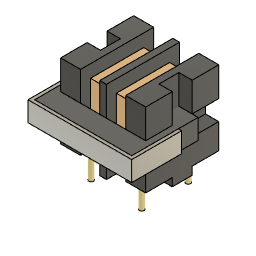
PowerLine_choke v2 (Autodesk Fusion 360 design; units mm, degrees)
Autodesk Fusion 360 part; units mm, degrees
note: some values were not read from the file. Chosen so that the rebuilt part matches the saved one: which bodies a step acts on.
sketch "Sketch1" plane through (0, 0, 0) normal (0, 0, 1) x (1, 0, 0) in component "PowerLine_choke"
  line L0 (10.2, -2) -> (10.2, 9)
  line L1 (-2.6, 9) -> (-2.6, -2)
  line L2 (7.2, 9) -> (7.2, -2)
  line L3 (0.4, 9) -> (0.4, -2)
  circle A0 centre (0, 7) radius 0.35
  circle A1 centre (7.62, 7) radius 0.35
  circle A2 centre (0, 0) radius 0.35
  circle A3 centre (7.62, 0) radius 0.35
  line L4 (3.3, 9) -> (3.3, -2)
  line L5 (4.3, -2) -> (4.3, 9)
  line L6 (0.4, 9) -> (-2.6, 9)
  line L7 (10.2, 9) -> (7.2, 9)
  line L8 (4.3, 9) -> (3.3, 9)
  line L9 (7.2, -2) -> (10.2, -2)
  line L10 (-2.6, -2) -> (0.4, -2)
  line L11 (3.3, -2) -> (4.3, -2)
  line L12 (7.2, -0.5) -> (4.3, -0.5)
  line L13 (3.3, -0.5) -> (0.4, -0.5)
  line L14 (0.4, 7.5) -> (3.3, 7.5)
  line L15 (4.3, 7.5) -> (7.2, 7.5)
  line L16 (10.2, 2) -> (8.2, 2)
  line L17 (-0.6, 2) -> (-2.6, 2)
  line L18 (-2.6, 5) -> (-0.6, 5)
  line L19 (8.2, 5) -> (10.2, 5)
  line L20 (8.2, 5) -> (8.2, 2)
  line L21 (-0.6, 5) -> (-0.6, 2)
  line L22 (-0.6, 5) -> (8.2, 5)
  line L23 (8.2, 2) -> (-0.6, 2)
  line L24 (-0.6, 5) -> (-0.6, 9)
  line L25 (-0.6, 2) -> (-0.6, -2)
  line L26 (8.2, 2) -> (8.2, -2)
  line L27 (8.2, 5) -> (8.2, 9)
  dimension "d1" = 7.62
  dimension "d2" = 7
  dimension "d3" = 12.8
  dimension "d4" = 11
  dimension "d6" = 3
  dimension "d7" = 0.7
  dimension "d8" = 0.7
  dimension "d9" = 0.7
  dimension "d10" = 0.7
  constraint horizontal L10
  constraint vertical L0
  constraint horizontal L7
  constraint vertical L1
  constraint coincident L2.end L10
  constraint perpendicular L2 L10
  constraint perpendicular L3 L10
  constraint coincident L3.start L7
  constraint coincident A2.centre origin
  constraint collinear L6 L7
  constraint collinear L7 L8
  constraint collinear L9 L10
  constraint collinear L10 L11
  constraint horizontal L14
  constraint horizontal L12
  constraint coincident L2 L12.start
  constraint coincident L2 L15.end
  constraint coincident L3 L14.start
  constraint coincident L3 L13.end
  constraint coincident L5 L12.end
  constraint coincident L4 L13.start
  constraint collinear L12 L13
  constraint coincident L4 L14.end
  constraint coincident L5 L15.start
  constraint collinear L14 L15
  constraint horizontal L18
  constraint horizontal L16
  constraint coincident L1 L18.start
  constraint coincident L1 L17.end
  constraint coincident L0 L19.end
  constraint coincident L0 L16.start
  constraint collinear L16 L17
  constraint collinear L18 L19
  constraint perpendicular L16 L20
  constraint perpendicular L17 L21
  constraint perpendicular L20 L22
  constraint perpendicular L21 L23
  constraint coincident L6 L24.end
  constraint perpendicular L6 L24
  constraint perpendicular L23 L25
  constraint coincident L9 L26.end
  constraint perpendicular L9 L26
  constraint coincident L7 L27.end
  constraint perpendicular L7 L27
  measures "d1" distance of A2.centre A3.centre
  measures "d2" distance of A2.centre A0.centre
  measures "d3" distance of L1.end L0.start
  measures "d4" distance of L1.end L1.start
  measures "d6" distance of L1 L3
  measures "d7" diameter of A0
  measures "d8" diameter of A1
  measures "d9" diameter of A2
  measures "d10" diameter of A3
extrude "Extrude1" add sketch "Sketch1" along normal blind 12.4 contours L0 L9 L16 L26 | L2 L9 L23 L26 | L0 L7 L19 L27 | L2 L20 L22 L23 | L2 L7 L22 L27 | L4 L5 L22 L23 | L4 L5 L11 L23 | L4 L5 L8 L22 | L3 L21 L22 L23 | L3 L10 L23 L25 | L3 L6 L22 L24 | L1 L10 L17 L25 | L1 L6 L18 L24 | A0 | A1 | A2 | A3 makes body 1 at (0.4, 5.3333, 4.1333) makes body 2 at (7.2, 5.3333, 4.1333) makes body 3 at (4.3, 1.6667, 4.1333) in component "PowerLine_choke"
extrude "Extrude2" cut sketch "Sketch1" along normal blind 1.2 contours L0 L9 L16 L26 | L2 L9 L23 L26 | L0 L7 L19 L27 | L2 L20 L22 L23 | L2 L7 L22 L27 | L3 L21 L22 L23 | L3 L10 L23 L25 | L3 L6 L22 L24 | L1 L10 L17 L25 | L1 L6 L18 L24 | A0 | A1 | A2 | A3 bodies 1 2 in component "PowerLine_choke"
extrude "Extrude3" add sketch "Sketch1" along normal blind 5 contours L0 L16 L19 L20 | L1 L17 L18 L21 bodies 1 2 in component "PowerLine_choke"
extrude "Extrude4" add sketch "Sketch1" along normal blind 8 and the other way blind -6 contours L2 L5 L22 L23 | L3 L4 L22 L23 bodies 1 2 3 in component "PowerLine_choke"
extrude "Extrude5" cut sketch "Sketch1" along normal blind 5 and the other way blind -8 contours L0 L9 L16 L26 | L0 L7 L19 L27 | L1 L10 L17 L25 | L1 L6 L18 L24 bodies 1 in component "PowerLine_choke"
sketch "Sketch2" plane through (0, 0, 0) normal (0, 0, 1) x (1, 0, 0) in component "PowerLine_choke"
  line L0 (-3.5, 5) -> (11.1, 5)
  line L1 (11.1, 5) -> (11.1, -5)
  line L2 (11.1, -5) -> (-3.5, -5)
  line L3 (-3.5, -5) -> (-3.5, 5)
  line L4 (8.2, 2) -> (-0.6, 2)
  line L5 (-0.6, 2) -> (-0.6, -2)
  line L6 (-0.6, -2) -> (8.2, -2)
  line L7 (8.2, -2) -> (8.2, 2)
  line L8 (11.6, 2) -> (11.6, -5.5)
  line L9 (11.6, -5.5) -> (-4, -5.5)
  line L10 (-4, -5.5) -> (-4, 2)
  line L11 (-4, 2) -> (-3.5, 2)
  line L12 (11.1, 2) -> (11.6, 2)
  dimension "d27" = 14.6
  dimension "d28" = 10
  constraint horizontal L0
  constraint vertical L1
  constraint horizontal L2
  constraint vertical L3
  constraint horizontal L4
  constraint perpendicular L4 L5
  constraint perpendicular L5 L6
  constraint perpendicular L4 L7
  constraint horizontal L11
  constraint vertical L8
  constraint horizontal L9
  constraint vertical L10
  constraint coincident L1 L12.start
  constraint collinear L11 L12
  constraint coincident L3 L11.end
  measures "d27" distance of L0.start L0.end
  measures "d28" distance of L0.start L2.end
extrude "Extrude6" add sketch "Sketch2" along normal blind 8 and the other way blind -5 separate body contours L0 L1 L2 L3 makes body 4 in component "PowerLine_choke"
extrude "Extrude7" add sketch "Sketch2" along normal blind 8 and the other way blind -5 separate body contours L1 L2 L3 L8 L9 L10 L11 L12 makes body 5 in component "PowerLine_choke"
sketch "Sketch3" plane through (0, 0, 0) normal (0, 0, 1) x (1, 0, 0) in component "PowerLine_choke"
extrude "Extrude8" add sketch "Sketch1" along normal blind 10.5 and the other way blind -3 separate body contours L2 L5 L22 L23 | L2 L5 L12 L23 | L2 L5 L15 L22 | L3 L4 L22 L23 | L3 L4 L13 L23 | L3 L4 L14 L22 makes body 6 at (0.4, 4.8333, 5.5) makes body 7 at (4.3, 2.1667, 5.5) in component "PowerLine_choke"
extrude "Extrude9" add sketch "Sketch1" along normal blind 1.2 and the other way blind 3.2 separate body contours A0 | A1 | A2 | A3 makes body 8 at (7.9683, -0.0348, -2.1333) makes body 9 at (7.9683, 6.9652, -2.1333) makes body 10 at (0.3483, -0.0348, -2.1333) makes body 11 at (0.3483, 6.9652, -2.1333) in component "PowerLine_choke"
component "PowerLine_choke" placed x (1, 0, 0) y (0, 1, 0) z (0, 0, 1) at (0, 0, 0)
equation "d1 = ( 2.54 * 3 ) * 1 mm"
named bodies: "Plastic", "Core", "metal_clip", "winding1", "winding2", "pin2", "pin4", "pin1", "pin3"
